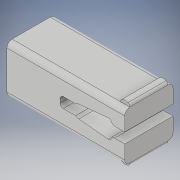
# Autodesk Inventor part: Connector_pin_stick
Saved by Autodesk Inventor 2019.3 (Build 233278000, 278)
## iProperties
Created: 2019-02-05
Part Number: Connector_pin_stick
Material: Generic
Document SubType Name: Modeling
Designer: Varga Daniel
Density: 1 g/cm^3
Appearance: Default
Author: Varga Daniel
Autodesk Inventor part; units mm, degrees
ref_plane "YZ Plane" through (0, 0, 0) normal (1, 0, 0) x (0, 1, 0)
ref_plane "XZ Plane" through (0, 0, 0) normal (0, 1, 0) x (-1, 0, 0)
ref_plane "XY Plane" through (0, 0, 0) normal (0, 0, 1) x (1, 0, 0)
derived "Connector_pin_base.ipt"
sketch "Pin_base_sketch" plane through (0, 0, 0) normal (0, 0, 1) x (1, 0, 0)
  line L0 (0, 0) -> (23.0918, 0) construction
  line L1 (0, 0) -> (0, 6.22) construction
  line L2 (0, 3.75) -> (0.563, 3.75)
  line L3 (0.863, 3.45) -> (0.863, 2.475)
  line L4 (0.863, 2.475) -> (9.988, 2.475)
  line L5 (9.988, 2.475) -> (9.988, 0)
  line L6 (0, 0) -> (0, 3.75)
  line L7 (0, 0) -> (9.988, 0)
  line L8 (9.288, 2.475) -> (9.288, 2.6)
  line L9 (9.988, 2.475) -> (9.988, 2.4774)
  arc A0 (9.988, 2.4774) -> (9.8454, 2.7031) centre (9.738, 2.4774) ccw
  arc A1 (9.8454, 2.7031) -> (9.288, 2.6) centre (9.6379, 2.267) ccw
  line L10 (9.8454, 2.7031) -> (9.8454, -0.0362) construction
  line L11 (8.9584, 2.75) -> (10.3858, 2.75) construction
  arc A2 (0.863, 3.45) -> (0.563, 3.75) centre (0.563, 3.45) ccw
  line L12 (0.863, 2.475) -> (0.863, 0)
  line L13 (-0.863, 2.475) -> (-0.863, 0)
  line L14 (-0.863, 3.45) -> (-0.863, 2.475)
  arc A3 (-0.563, 3.75) -> (-0.863, 3.45) centre (-0.563, 3.45) ccw
  line L15 (0, 3.75) -> (-0.563, 3.75)
  line L16 (0, 0) -> (-23.0918, 0) construction
  line L17 (0, 0) -> (-9.988, 0)
  line L18 (-0.863, 2.475) -> (-9.988, 2.475)
  line L19 (-9.288, 2.475) -> (-9.288, 2.6)
  arc A4 (-9.288, 2.6) -> (-9.8454, 2.7031) centre (-9.6379, 2.267) ccw
  arc A5 (-9.8454, 2.7031) -> (-9.988, 2.4774) centre (-9.738, 2.4774) ccw
  line L20 (-9.988, 2.475) -> (-9.988, 2.4774)
  line L21 (-8.9584, 2.75) -> (-10.3858, 2.75) construction
  line L22 (-9.8454, 2.7031) -> (-9.8454, -0.0362) construction
  line L23 (-9.988, 2.475) -> (-9.988, 0)
  line L24 (9.638, 3.1946) -> (9.638, -1.2485) construction
  dimension "d7" = 9.125
  measures "d7" distance between parallel lines of L5 L12
sketch "Pin_hole_sketch" plane through (0, 0, 0) normal (0, 0, 1) x (1, 0, 0)
  line L0 (0, 0) -> (23.0918, 0) construction
  line L1 (9.988, 2.475) -> (9.988, 0) construction
  line L2 (9.988, 0.4) -> (9.206, 0.4)
  line L3 (9.988, 0.4) -> (9.988, 0)
  line L4 (9.988, 0) -> (4.988, 0)
  line L5 (8.7138, 0.722) -> (6.4388, 0.498)
  arc A0 (8.9722, 0.5616) -> (8.7138, 0.722) centre (8.7383, 0.4732) ccw
  arc A1 (8.9722, 0.5616) -> (9.206, 0.4) centre (9.206, 0.65) ccw
  line L6 (4.988, 0) -> (4.988, 0.15)
  line L7 (5.238, 0.4) -> (6.1873, 0.4)
  arc A2 (5.238, 0.4) -> (4.988, 0.15) centre (5.238, 0.15) ccw
  arc A3 (6.4388, 0.498) -> (6.1873, 0.4) centre (6.4878, 0.0004) ccw
  line L8 (0, 0) -> (0, 6.22) construction
  arc A4 (-6.1873, 0.4) -> (-6.4388, 0.498) centre (-6.4878, 0.0004) ccw
  line L9 (-5.238, 0.4) -> (-6.1873, 0.4)
  line L10 (-4.988, 0) -> (-4.988, 0.15)
  arc A5 (-4.988, 0.15) -> (-5.238, 0.4) centre (-5.238, 0.15) ccw
  line L11 (-8.7138, 0.722) -> (-6.4388, 0.498)
  line L12 (-9.988, 0) -> (-4.988, 0)
  arc A6 (-8.7138, 0.722) -> (-8.9722, 0.5616) centre (-8.7383, 0.4732) ccw
  arc A7 (-9.206, 0.4) -> (-8.9722, 0.5616) centre (-9.206, 0.65) ccw
  line L13 (-9.988, 2.475) -> (-9.988, 0) construction
  line L14 (-9.988, 0.4) -> (-9.206, 0.4)
  line L15 (-9.988, 0.4) -> (-9.988, 0)
  arc A8 (6.1873, -0.4) -> (6.4388, -0.498) centre (6.4878, -0.0004) ccw
  line L16 (8.7138, -0.722) -> (6.4388, -0.498)
  arc A9 (8.7138, -0.722) -> (8.9722, -0.5616) centre (8.7383, -0.4732) ccw
  arc A10 (9.206, -0.4) -> (8.9722, -0.5616) centre (9.206, -0.65) ccw
  line L17 (9.988, -2.475) -> (9.988, 0) construction
  line L18 (9.988, -0.4) -> (9.206, -0.4)
  line L19 (9.988, -0.4) -> (9.988, 0)
  line L20 (4.988, 0) -> (4.988, -0.15)
  arc A11 (4.988, -0.15) -> (5.238, -0.4) centre (5.238, -0.15) ccw
  arc A12 (-5.238, -0.4) -> (-4.988, -0.15) centre (-5.238, -0.15) ccw
  line L21 (-5.238, -0.4) -> (-6.1873, -0.4)
  line L22 (5.238, -0.4) -> (6.1873, -0.4)
  line L23 (-4.988, 0) -> (-4.988, -0.15)
  arc A13 (-6.4388, -0.498) -> (-6.1873, -0.4) centre (-6.4878, -0.0004) ccw
  line L24 (-8.7138, -0.722) -> (-6.4388, -0.498)
  arc A14 (-8.9722, -0.5616) -> (-8.7138, -0.722) centre (-8.7383, -0.4732) ccw
  arc A15 (-8.9722, -0.5616) -> (-9.206, -0.4) centre (-9.206, -0.65) ccw
  line L25 (-9.988, -0.4) -> (-9.206, -0.4)
  line L26 (-9.988, -0.4) -> (-9.988, 0)
  line L27 (-9.988, -2.475) -> (-9.988, 0) construction
derived "Base_part.ipt"
sketch "Axle_sketch" plane through (0, 0, 0) normal (0, 1, 0) x (-1, 0, 0)
  circle A0 centre (-15.8957, 4.3197) radius 2.5 construction
  line L0 (-14.4207, 2.4447) -> (-17.3707, 2.4447)
  line L1 (-17.7707, 2.8447) -> (-17.7707, 5.7947)
  line L2 (-17.3707, 6.1947) -> (-14.4207, 6.1947)
  line L3 (-14.0207, 5.7947) -> (-14.0207, 2.8447)
  line L4 (-14.0207, 2.4447) -> (-17.7707, 6.1947) construction
  line L5 (-17.7707, 2.4447) -> (-14.0207, 6.1947) construction
  arc A1 (-14.4207, 2.4447) -> (-14.0207, 2.8447) centre (-14.4207, 2.8447) ccw
  arc A2 (-17.7707, 2.8447) -> (-17.3707, 2.4447) centre (-17.3707, 2.8447) ccw
  arc A3 (-14.0207, 5.7947) -> (-14.4207, 6.1947) centre (-14.4207, 5.7947) ccw
  arc A4 (-17.3707, 6.1947) -> (-17.7707, 5.7947) centre (-17.3707, 5.7947) ccw
  point P0 (0, 0)
  dimension "d9" = 3.75
  dimension "d10" = 0.4
  dimension "d11" = 3.75
  measures "d9" distance between parallel lines of L3 L1
  measures "d10" radius of A2
  measures "d11" distance between parallel lines of L0 L2
sketch "Sketch5" plane through (0, 0, 0) normal (0, 0, 1) x (1, 0, 0)
  line L0 (0.863, 2.475) -> (0.863, 0) projected
  line L1 (9.988, 2.475) -> (9.988, 0) construction
  line L2 (0.863, 2.475) -> (9.988, 2.475) construction
  line L3 (9.288, 2.475) -> (9.288, 2.6) construction
  arc A0 (9.8454, 2.7031) -> (9.288, 2.6) centre (9.6379, 2.267) ccw construction
  arc A1 (9.988, 2.4774) -> (9.8454, 2.7031) centre (9.738, 2.4774) ccw construction
  line L4 (9.988, 2.475) -> (9.988, 2.4774) construction
  line L5 (9.988, 2.475) -> (9.988, 0) projected
  line L6 (0, 0) -> (23.0918, 0) construction
  line L7 (0.863, 2.475) -> (9.988, 2.475) construction
  line L8 (9.988, 2.4774) -> (9.988, 2.475) construction
  line L9 (9.288, 2.475) -> (9.288, 2.6) construction
  arc A2 (9.8454, 2.7031) -> (9.288, 2.6) centre (9.6379, 2.267) ccw construction
  arc A3 (9.988, 2.4774) -> (9.8454, 2.7031) centre (9.738, 2.4774) ccw construction
  line L10 (0.863, 1.875) -> (9.988, 1.875)
  line L11 (9.988, 1.8774) -> (9.988, 1.875)
  line L12 (9.288, 1.875) -> (9.288, 2)
  arc A4 (9.8454, 2.1031) -> (9.288, 2) centre (9.6379, 1.667) ccw
  arc A5 (9.988, 1.8774) -> (9.8454, 2.1031) centre (9.738, 1.8774) ccw
  line L13 (9.988, 1.8774) -> (9.988, 0)
  line L14 (9.988, 0) -> (0.863, 0)
  line L15 (0.863, 0) -> (0.863, 1.875)
  line L16 (0.863, -1.875) -> (9.988, -1.875)
  line L17 (9.988, -1.8774) -> (9.988, -1.875)
  line L18 (9.288, -1.875) -> (9.288, -2)
  arc A6 (9.288, -2) -> (9.8454, -2.1031) centre (9.6379, -1.667) ccw
  arc A7 (9.8454, -2.1031) -> (9.988, -1.8774) centre (9.738, -1.8774) ccw
  line L19 (9.988, -1.8774) -> (9.988, 0)
  line L20 (0.863, 0) -> (0.863, -1.875)
  point P0 (9.6379, -2.267)
  point P1 (9.6379, -2.267)
  dimension "d14" = 0.6
  dimension "d19" = 4.95
  dimension "d20" = 3.75
  constraints: 28 end point, 12 point on circle, 10 symmetric about line, 6 centre point, 4 point on line, 2 collinear, 2 concentric, 2 perpendicular, 1 vertical, 15 other
  measures "d14" distance of L0.start L10.start
  measures "d19" diameter of L2 L6
  measures "d20" diameter of L10 L6
extrude "Extrusion3" add sketch "Sketch5" along normal mid plane 3.75
extrude "Extrusion4" cut sketch "Pin_hole_sketch" along normal through all both and the other way through all contours L3 L4 L6 A2 L7 A3 L5 A0 A1 L2 | L19 L18 A10 A9 L16 A8 L22 A11 L20 L4
fillet "Fillet1" radius 0.4 4 edges at (5.0755, -1.875, 1.875) (5.0755, -1.875, -1.875) (5.0755, 1.875, 1.875) (5.0755, 1.875, -1.875)
sketch "Sketch8" plane through (9.288, 2, -1.875) normal (-1, 0, 0) x (0, 0, 1)
  arc A0 (0.4, -0.125) -> (0, -0.525) centre (0.4, -0.525) ccw projected
  line L0 (0, -3.475) -> (0, -0.525) projected
  arc A1 (0, -3.475) -> (0.4, -3.875) centre (0.4, -3.475) ccw projected
  line L1 (0.4, -3.875) -> (3.35, -3.875) projected
  arc A2 (3.35, -3.875) -> (3.75, -3.475) centre (3.35, -3.475) ccw projected
  line L2 (3.75, -0.525) -> (3.75, -3.475) projected
  arc A3 (3.75, -0.525) -> (3.35, -0.125) centre (3.35, -0.525) ccw projected
  line L3 (0.4, -0.125) -> (3.35, -0.125) projected
  line L4 (0, -0.525) -> (0, 1.475)
  line L5 (0, 1.475) -> (0.4, 1.475)
  line L6 (0.4, 1.475) -> (0.4, -0.125)
  line L7 (3.75, -0.5584) -> (3.75, 1.475)
  line L8 (3.75, 1.475) -> (3.35, 1.475)
  line L9 (3.35, 1.475) -> (3.35, -0.125)
  line L10 (3.75, -3.475) -> (3.75, -5.475)
  line L11 (3.75, -5.475) -> (3.35, -5.475)
  line L12 (3.35, -5.475) -> (3.35, -3.875)
  line L13 (0.4, -3.875) -> (0.4, -5.475)
  line L14 (0.4, -5.475) -> (0, -5.475)
  line L15 (0, -3.475) -> (0, -5.475)
  point P0 (1.875, -2)
  dimension "d27" = 2
  dimension "d30" = 2
  constraints: 24 end point, 5 collinear, 4 parallel, 3 perpendicular, 1 point on line
  measures "d27" distance from line of L0.end L5
  measures "d30" distance from line of L0.start L14
extrude "Extrusion6" cut sketch "Sketch8" against normal through all contours A0 L4 L5 L6 | L9 L8 L7 A3 | A1 L13 L14 L15 | A2 L10 L11 L12
ref_plane "Work Plane1" through (0.863, 0, -1.475) normal (0, -1, 0) x (1, 0, 0)
ref_plane "Work Plane2" through (0, 0, 0) normal (0, 0, -1) x (-1, 0, 0)
equation "\"d14\" = -0.5 * d9 + 0.5 * d19"
equation "\"d21\" = d9"
equation "\"d25\" = d10"
equation "\"d30\" = d27"
body "Solid3"
